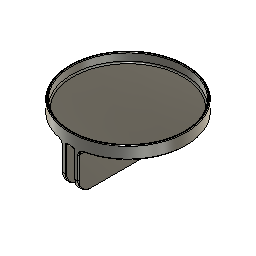
FRESHER-STAND (Autodesk Fusion 360 design; units mm, degrees)
Autodesk Fusion 360 part; units mm, degrees
sketch "Sketch1" plane through (0, 0, 0) normal (0, 0, 1) x (1, 0, 0)
  circle A0 centre (0, 0) radius 45
  dimension "d1" = 90
  constraint coincident A0.centre origin
  measures "d1" diameter of A0
extrude "Extrude1" add sketch "Sketch1" along normal blind 10
sketch "Sketch2" plane through (0, 0, 10) normal (0, 0, 1) x (-1, 0, 0)
  circle A0 centre (0, 0) radius 45
  circle A1 centre (0, 0) radius 43.5
  dimension "d4" = 87
  constraint coincident A0.centre A1.centre
  measures "d4" diameter of A1
extrude "Extrude2" cut sketch "Sketch2" against normal blind 7 contours A1
sketch "Sketch6" plane through (0, 0, 0) normal (0, 0, -1) x (1, 0, 0)
  circle A0 centre (0, 0) radius 45
  line L0 (-3.25, 50) -> (-6.25, 50)
  line L1 (-6.25, 50) -> (-6.25, -50)
  line L2 (-6.25, -50) -> (-3.25, -50)
  line L3 (-3.25, -50) -> (-3.25, 50)
  line L4 (3.25, 50) -> (6.25, 50)
  line L5 (6.25, 50) -> (6.25, -50)
  line L6 (6.25, -50) -> (3.25, -50)
  line L7 (3.25, -50) -> (3.25, 50)
  dimension "d16" = 3
  dimension "d17" = 3
  dimension "d18" = 3.25
  dimension "d19" = 3.25
  constraint horizontal L0
  constraint vertical L1
  constraint horizontal L2
  constraint vertical L3
  constraint horizontal L4
  constraint vertical L5
  constraint horizontal L6
  constraint vertical L7
  measures "d16" distance of L1.end L2.end
  measures "d17" distance of L5.end L6.end
  measures "d18" distance of A0.centre L3
  measures "d19" distance of A0.centre L7
extrude "Extrude3" add sketch "Sketch6" along normal blind 30 contours A0 L5 L7 | A0 L1 L3
fillet "Fillet1" radius 10 4 edges at (4.7527, -44.7483, -30) (-4.7527, -44.7483, -30) (4.7527, 44.7483, -30) (-4.7527, 44.7483, -30)
fillet "Fillet2" radius 1 4 edges at (45, 0, 0) (0, -45, 0) (-45, 0, 0) (0, 45, 0)
fillet "Fillet3" radius 3 6 edges at (6.25, -44.2665, 0.2913) (6.25, 0, 0) (6.25, 44.2665, 0.2913) (-6.25, 44.2665, 0.2913) (-6.25, 0, 0) (-6.25, -44.2665, 0.2913)
fillet "Fillet4" radius 1 6 edges at (-3.25, -44.5884, 0.2925) (-3.25, 0, 0) (-3.25, 44.5884, 0.2925) (3.25, 44.5884, 0.2925) (3.25, 0, 0) (3.25, -44.5884, 0.2925)
fillet "Fillet5" radius 0.5 28 edges at (7.0199, 44.4491, -0.4446) (6.25, 44.5639, -11.3513) (6.25, 41.5809, -27.094) (6.25, 0, -30) (6.25, -41.5809, -27.094) (6.25, -44.5639, -11.3513) (7.0199, -44.4491, -0.4446) (2.8815, -44.9076, 0.2438) (3.25, -44.8825, -10.383) (3.25, -41.9392, -27.0772) (3.25, 0, -30) (3.25, 41.9392, -27.0772) (3.25, 44.8825, -10.383) (2.8815, 44.9076, 0.2438) (-2.8815, 44.9076, 0.2438) (-3.25, 44.8825, -10.383) (-3.25, 41.9392, -27.0772) (-3.25, 0, -30) (-3.25, -41.9392, -27.0772) (-3.25, -44.8825, -10.383) (-2.8815, -44.9076, 0.2438) (-7.0199, -44.4491, -0.4446) (-6.25, -44.5639, -11.3513) (-6.25, -41.5809, -27.094) (-6.25, 0, -30) (-6.25, 41.5809, -27.094) (-6.25, 44.5639, -11.3513) (-7.0199, 44.4491, -0.4446)
fillet "Fillet6" radius 1 1 edges at (40.5562, -15.7303, 3)
fillet "Fillet7" radius 0.5 2 edges at (40.5562, -15.7303, 10) (-41.9547, -16.2727, 10)
